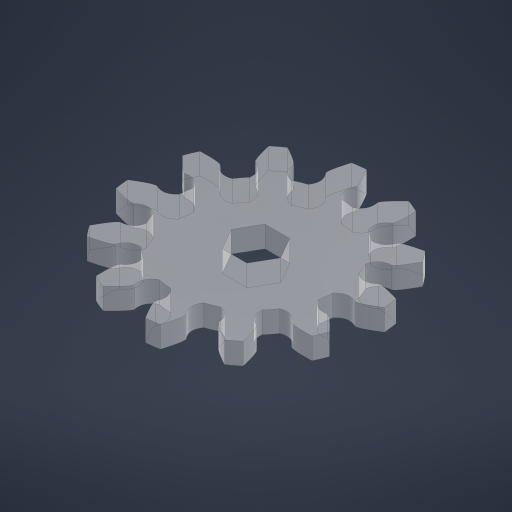
# Autodesk Inventor part: CORL_005_PolyCarbSprocket
Saved by Autodesk Inventor 2024.2 (Build 282272000, 272)
## iProperties
Created: 2024-08-02
Part Number: CORL_005_PolyCarbSprocket
Material: Polycarbonate, Clear
Document SubType Name: Modeling
Designer: Bryan
Density: 1.2 g/cm^3
Appearance: Polycarbonate - Clear
Author: Bryan
Autodesk Inventor part; units mm, degrees
ref_plane "YZ Plane" through (0, 0, 0) normal (1, 0, 0) x (0, 1, 0)
ref_plane "XZ Plane" through (0, 0, 0) normal (0, 1, 0) x (-1, 0, 0)
ref_plane "XY Plane" through (0, 0, 0) normal (0, 0, 1) x (1, 0, 0)
sketch "Sketch1" plane through (0, 0, 0) normal (0, 1, 0) x (-1, 0, 0)
  circle A0 centre (0, 0) radius 30.48 construction
  circle A1 centre (0, 0) radius 35.56
  circle A2 centre (0, 0) radius 24.13
  line L0 (0, 0) -> (0, -30.48) construction
  line L1 (0, -30.48) -> (7.3885, -28.5692) construction
  line L2 (7.3885, -28.5692) -> (0, 0) construction
  line L3 (18.2524, -23.1871) -> (2.6609, -35.4603) construction
  arc A3 (7.3885, -28.5692) -> (18.2524, -23.1871) centre (0, 0) ccw construction
  arc A4 (-0.1636, -29.5087) -> (7.3885, -28.5692) centre (0, 0) ccw construction
  line L4 (24.8198, -25.4655) -> (-27.3485, -22.7283) construction
  line L5 (-0.1636, -29.5087) -> (-1.2643, -24.0969) construction
  line L6 (13.9703, -32.7008) -> (-33.7032, -11.3405) construction
  line L7 (-0.1636, -29.5087) -> (0.3319, -26.5901) construction
  line L8 (0.3319, -26.5901) -> (-1.2643, -24.0969) construction
  spline S0 degree 2 poles (2.6609, -35.4603) (-0.3598, -30.6028) (-0.1636, -29.5087) knots 0 0 0 1 1 1
  spline S1 degree 2 poles (-0.1636, -29.5087) (1.3777, -26.3773) (-1.2643, -24.0969) knots 0 0 0 1 1 1
  line L9 (0, 0) -> (-3.1496, -23.9236) construction
  spline S2 degree 2 poles (-11.7481, -33.5633) (-7.573, -29.6531) (-7.4794, -28.5456) knots 0 0 0 1 1 1
  spline S3 degree 2 poles (-7.4794, -28.5456) (-8.1577, -25.122) (-5.0155, -23.603) knots 0 0 0 1 1 1
  spline S4 degree 2 poles (20.0346, -29.3791) (14.9898, -26.6827) (14.6126, -25.6371) knots 0 0 0 1 1 1
  spline S5 degree 2 poles (14.6126, -25.6371) (14.3818, -22.1546) (10.9535, -21.5007) knots 0 0 0 1 1 1
  spline S6 degree 2 poles (7.7955, -28.4609) (5.4962, -25.8351) (7.458, -22.9485) knots 0 0 0 1 1 1
  spline S7 degree 2 poles (6.6075, -34.9407) (8.2681, -29.4669) (7.7955, -28.4609) knots 0 0 0 1 1 1
  spline S8 degree 2 poles (32.04, -15.4257) (26.3229, -15.613) (25.4735, -14.896) knots 0 0 0 1 1 1
  spline S9 degree 2 poles (25.4735, -14.896) (23.5323, -11.9956) (20.2363, -13.1434) knots 0 0 0 1 1 1
  spline S10 degree 2 poles (20.9815, -20.7501) (17.6774, -19.6258) (17.9331, -16.145) knots 0 0 0 1 1 1
  spline S11 degree 2 poles (23.1927, -26.9558) (21.8938, -21.385) (20.9815, -20.7501) knots 0 0 0 1 1 1
  spline S12 degree 2 poles (35.4603, 2.6609) (30.6028, -0.3598) (29.5087, -0.1636) knots 0 0 0 1 1 1
  spline S13 degree 2 poles (29.5087, -0.1636) (26.3773, 1.3777) (24.0969, -1.2643) knots 0 0 0 1 1 1
  spline S14 degree 2 poles (28.5456, -7.4794) (25.122, -8.1577) (23.603, -5.0155) knots 0 0 0 1 1 1
  spline S15 degree 2 poles (33.5633, -11.7481) (29.6531, -7.573) (28.5456, -7.4794) knots 0 0 0 1 1 1
  spline S16 degree 2 poles (29.3791, 20.0346) (26.6827, 14.9898) (25.6371, 14.6126) knots 0 0 0 1 1 1
  spline S17 degree 2 poles (25.6371, 14.6126) (22.1546, 14.3818) (21.5007, 10.9535) knots 0 0 0 1 1 1
  spline S18 degree 2 poles (28.4609, 7.7955) (25.8351, 5.4962) (22.9485, 7.458) knots 0 0 0 1 1 1
  spline S19 degree 2 poles (34.9407, 6.6075) (29.4669, 8.2681) (28.4609, 7.7955) knots 0 0 0 1 1 1
  spline S20 degree 2 poles (15.4257, 32.04) (15.613, 26.3229) (14.896, 25.4735) knots 0 0 0 1 1 1
  spline S21 degree 2 poles (14.896, 25.4735) (11.9956, 23.5323) (13.1434, 20.2363) knots 0 0 0 1 1 1
  spline S22 degree 2 poles (20.7501, 20.9815) (19.6258, 17.6774) (16.145, 17.9331) knots 0 0 0 1 1 1
  spline S23 degree 2 poles (26.9558, 23.1927) (21.385, 21.8938) (20.7501, 20.9815) knots 0 0 0 1 1 1
  spline S24 degree 2 poles (-2.6609, 35.4603) (0.3598, 30.6028) (0.1636, 29.5087) knots 0 0 0 1 1 1
  spline S25 degree 2 poles (0.1636, 29.5087) (-1.3777, 26.3773) (1.2643, 24.0969) knots 0 0 0 1 1 1
  spline S26 degree 2 poles (7.4794, 28.5456) (8.1577, 25.122) (5.0155, 23.603) knots 0 0 0 1 1 1
  spline S27 degree 2 poles (11.7481, 33.5633) (7.573, 29.6531) (7.4794, 28.5456) knots 0 0 0 1 1 1
  spline S28 degree 2 poles (-20.0346, 29.3791) (-14.9898, 26.6827) (-14.6126, 25.6371) knots 0 0 0 1 1 1
  spline S29 degree 2 poles (-14.6126, 25.6371) (-14.3818, 22.1546) (-10.9535, 21.5007) knots 0 0 0 1 1 1
  spline S30 degree 2 poles (-7.7955, 28.4609) (-5.4962, 25.8351) (-7.458, 22.9485) knots 0 0 0 1 1 1
  spline S31 degree 2 poles (-6.6075, 34.9407) (-8.2681, 29.4669) (-7.7955, 28.4609) knots 0 0 0 1 1 1
  spline S32 degree 2 poles (-32.04, 15.4257) (-26.3229, 15.613) (-25.4735, 14.896) knots 0 0 0 1 1 1
  spline S33 degree 2 poles (-25.4735, 14.896) (-23.5323, 11.9956) (-20.2363, 13.1434) knots 0 0 0 1 1 1
  spline S34 degree 2 poles (-20.9815, 20.7501) (-17.6774, 19.6258) (-17.9331, 16.145) knots 0 0 0 1 1 1
  spline S35 degree 2 poles (-23.1927, 26.9558) (-21.8938, 21.385) (-20.9815, 20.7501) knots 0 0 0 1 1 1
  spline S36 degree 2 poles (-35.4603, -2.6609) (-30.6028, 0.3598) (-29.5087, 0.1636) knots 0 0 0 1 1 1
  spline S37 degree 2 poles (-29.5087, 0.1636) (-26.3773, -1.3777) (-24.0969, 1.2643) knots 0 0 0 1 1 1
  spline S38 degree 2 poles (-28.5456, 7.4794) (-25.122, 8.1577) (-23.603, 5.0155) knots 0 0 0 1 1 1
  spline S39 degree 2 poles (-33.5633, 11.7481) (-29.6531, 7.573) (-28.5456, 7.4794) knots 0 0 0 1 1 1
  spline S40 degree 2 poles (-29.3791, -20.0346) (-26.6827, -14.9898) (-25.6371, -14.6126) knots 0 0 0 1 1 1
  spline S41 degree 2 poles (-25.6371, -14.6126) (-22.1546, -14.3818) (-21.5007, -10.9535) knots 0 0 0 1 1 1
  spline S42 degree 2 poles (-28.4609, -7.7955) (-25.8351, -5.4962) (-22.9485, -7.458) knots 0 0 0 1 1 1
  spline S43 degree 2 poles (-34.9407, -6.6075) (-29.4669, -8.2681) (-28.4609, -7.7955) knots 0 0 0 1 1 1
  spline S44 degree 2 poles (-15.4257, -32.04) (-15.613, -26.3229) (-14.896, -25.4735) knots 0 0 0 1 1 1
  spline S45 degree 2 poles (-14.896, -25.4735) (-11.9956, -23.5323) (-13.1434, -20.2363) knots 0 0 0 1 1 1
  spline S46 degree 2 poles (-20.7501, -20.9815) (-19.6258, -17.6774) (-16.145, -17.9331) knots 0 0 0 1 1 1
  spline S47 degree 2 poles (-26.9558, -23.1927) (-21.385, -21.8938) (-20.7501, -20.9815) knots 0 0 0 1 1 1
  line L10 (3.6662, -6.35) -> (-3.6662, -6.35)
  line L11 (-3.6662, -6.35) -> (-7.3323, 0)
  line L12 (-7.3323, 0) -> (-3.6662, 6.35)
  line L13 (-3.6662, 6.35) -> (3.6662, 6.35)
  line L14 (3.6662, 6.35) -> (7.3323, 0)
  line L15 (7.3323, 0) -> (3.6662, -6.35)
  point P0 (-7.8888, -29.4414)
  point P1 (-7.2026, -25.5981)
  point P2 (15.24, -26.3965)
  point P3 (13.5824, -22.8617)
  point P4 (6.5615, -25.7699)
  point P5 (7.8888, -29.4414)
  point P6 (26.3965, -15.24)
  point P7 (23.1936, -13.0076)
  point P8 (18.5674, -19.0367)
  point P9 (21.5526, -21.5526)
  point P10 (30.48, 0)
  point P11 (26.5901, 0.3319)
  point P12 (25.5981, -7.2026)
  point P13 (29.4414, -7.8888)
  point P14 (26.3965, 15.24)
  point P15 (22.8617, 13.5824)
  point P16 (25.7699, 6.5615)
  point P17 (29.4414, 7.8888)
  point P18 (15.24, 26.3965)
  point P19 (13.0076, 23.1936)
  point P20 (19.0367, 18.5674)
  point P21 (21.5526, 21.5526)
  point P22 (0, 30.48)
  point P23 (-0.3319, 26.5901)
  point P24 (7.2026, 25.5981)
  point P25 (7.8888, 29.4414)
  point P26 (-15.24, 26.3965)
  point P27 (-13.5824, 22.8617)
  point P28 (-6.5615, 25.7699)
  point P29 (-7.8888, 29.4414)
  point P30 (-26.3965, 15.24)
  point P31 (-23.1936, 13.0076)
  point P32 (-18.5674, 19.0367)
  point P33 (-21.5526, 21.5526)
  point P34 (-30.48, 0)
  point P35 (-26.5901, -0.3319)
  point P36 (-25.5981, 7.2026)
  point P37 (-29.4414, 7.8888)
  point P38 (-26.3965, -15.24)
  point P39 (-22.8617, -13.5824)
  point P40 (-25.7699, -6.5615)
  point P41 (-29.4414, -7.8888)
  point P42 (-15.24, -26.3965)
  point P43 (-13.0076, -23.1936)
  point P44 (-19.0367, -18.5674)
  point P45 (-21.5526, -21.5526)
  point P46 (22.9485, 7.458)
  point P47 (29.3791, 20.0346)
  point P48 (26.9558, 23.1927)
  point P49 (16.145, 17.9331)
  point P50 (13.1434, 20.2363)
  point P51 (15.4257, 32.04)
  point P52 (11.7481, 33.5633)
  point P53 (5.0155, 23.603)
  point P54 (-2.6609, 35.4603)
  point P55 (-6.6075, 34.9407)
  point P56 (-7.458, 22.9485)
  point P57 (-10.9535, 21.5007)
  point P58 (-20.0346, 29.3791)
  point P59 (-23.1927, 26.9558)
  point P60 (-17.9331, 16.145)
  point P61 (-32.04, 15.4257)
  point P62 (-33.5633, 11.7481)
  point P63 (-23.603, 5.0155)
  point P64 (-35.4603, -2.6609)
  point P65 (-34.9407, -6.6075)
  point P66 (-22.9485, -7.458)
  point P67 (-29.3791, -20.0346)
  point P68 (-26.9558, -23.1927)
  point P69 (-16.145, -17.9331)
  point P70 (-13.1434, -20.2363)
  point P71 (-15.4257, -32.04)
  point P72 (-11.7481, -33.5633)
  point P73 (-5.0155, -23.603)
  point P74 (-1.2643, -24.0969)
  point P75 (6.6075, -34.9407)
  point P76 (7.458, -22.9485)
  point P77 (20.0346, -29.3791)
  point P78 (23.1927, -26.9558)
  point P79 (17.9331, -16.145)
  point P80 (32.04, -15.4257)
  point P81 (33.5633, -11.7481)
  point P82 (23.603, -5.0155)
  point P83 (35.4603, 2.6609)
  dimension "d18" = 60.96
  dimension "d19" = 71.12
  dimension "d20" = 48.26
  dimension "d21" = 14.5
  dimension "d22" = 7.6316
  dimension "d23" = 7.6316
  dimension "d24" = 19.8425
  dimension "d25" = 12.2109
  dimension "d27" = 75.5
  dimension "d28" = 75.5
  dimension "d29" = 7.5
  dimension "d32" = 360
  dimension "d34" = 12.7
  constraints: 32 end point, 5 point on circle, 5 symmetric about line, 4 coincident, 2 centre point, 1 equal length, 1 horizontal, 1 midpoint, 1 perpendicular, 1 point on line, 1 tangent, 1 vertical, 1 vertical alignment, 342 other
  measures "d21" angle of L0 L2
  measures "d22" distance of L0.end L1.end
  measures "d24" distance of L3.start L3.end
  measures "d27" angle of L4 L5
  measures "d28" angle of L6 L7
  measures "d29" angle of L9 L0
  measures "d34" distance between parallel lines of L13 L10
extrude "Extrusion1" add sketch "Sketch1" along normal blind 6.35 contours S12 S13 A2 S18 S19 A1 | A1 S8 S9 A2 S14 S15 | S16 S17 A2 S22 S23 A1 | A2 | A1 S4 S5 A2 S10 S11 | S20 S21 A2 S26 S27 A1 | A1 S0 S1 A2 S6 S7 | S24 S25 A2 S30 S31 A1 | A1 S44 S45 A2 S3 S2 | S28 S29 A2 S34 S35 A1 | A1 S40 S41 A2 S46 S47 | S32 S33 A2 S38 S39 A1 | A1 S36 S37 A2 S42 S43
equation "\"d18\" = PD"
equation "\"d19\" = OD"
equation "\"d20\" = RD"
equation "\"d21\" = a"
equation "\"d23\" = d22"
equation "\"d25\" = d24 - d22"
equation "\"PD\" = 60.96"
equation "\"a\" = 14.5deg"
equation "\"ded\" = 1.25 * mod"
equation "\"RD\" = PD - 2 * ded"
equation "\"OD\" = PD + 2 * mod"
equation "\"mod\" = 5.08"
body "Solid1"
